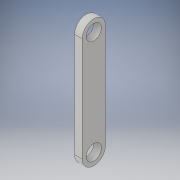
# Autodesk Inventor part: RollerArm
Saved by Autodesk Inventor 2017 (Build 210142000, 142)
## iProperties
Created: 2017-04-15
Part Number: RollerArm
Material: Generic
Document SubType Name: Modeling
Designer: User
Density: 1 g/cm^3
Appearance: Default
Author: User
Autodesk Inventor part; units mm, degrees
ref_plane "YZ Plane" through (0, 0, 0) normal (1, 0, 0) x (0, 1, 0)
ref_plane "XZ Plane" through (0, 0, 0) normal (0, 1, 0) x (-1, 0, 0)
ref_plane "XY Plane" through (0, 0, 0) normal (0, 0, 1) x (1, 0, 0)
sketch "Sketch1" plane through (0, 0, 0) normal (1, 0, 0) x (0, 1, 0)
  circle A0 centre (0, 0) radius 6.35
  arc A1 (0, 9.779) -> (0, -9.779) centre (0, 0) ccw
  line L0 (0, 9.779) -> (87.249, 9.779)
  line L1 (0, -9.779) -> (87.249, -9.779)
  arc A2 (87.249, -9.779) -> (87.249, 9.779) centre (87.249, 0) ccw
  circle A3 centre (87.249, 0) radius 6.35
  dimension "d0" = 12.7
  dimension "d1" = 19.558
  dimension "d2" = 87.249
  dimension "d3" = 87.249
  dimension "d4" = 12.7
  constraints: 4 centre point, 4 end point, 4 point on circle, 3 coincident, 3 tangent, 2 horizontal
  measures "d0" diameter of A0
  measures "d1" diameter of A1
  measures "d2" distance of L0.start L0.end
  measures "d3" distance of L1.start L1.end
  measures "d4" diameter of A3
extrude "Extrusion1" add sketch "Sketch1" along normal blind 6.35
body "Solid1"
